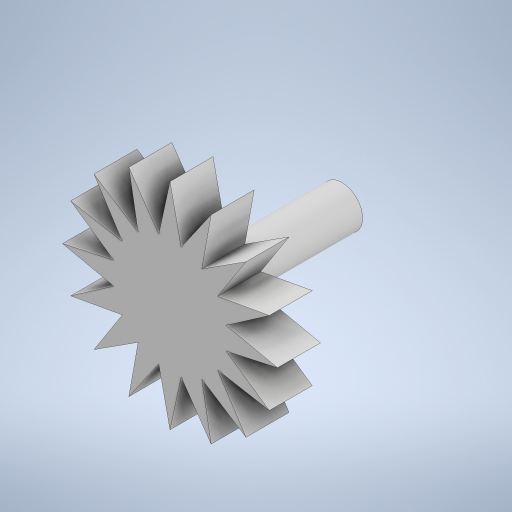
# Autodesk Inventor part: GEAR
Saved by Autodesk Inventor 2024.3 (Build 283343000, 343)
## iProperties
Created: 2024-07-29
Part Number: GEAR
Material: Ogólny
Document SubType Name: Modeling
Designer: User
Density: 1 g/cm^3
Appearance: Domyślna
Author: User
Autodesk Inventor part; units mm, degrees
ref_plane "YZ Plane" through (0, 0, 0) normal (1, 0, 0) x (0, 1, 0)
ref_plane "XZ Plane" through (0, 0, 0) normal (0, 1, 0) x (-1, 0, 0)
ref_plane "XY Plane" through (0, 0, 0) normal (0, 0, 1) x (1, 0, 0)
sketch "Szkic1" plane through (0, 0, 0) normal (0, 0, 1) x (1, 0, 0)
  circle A0 centre (0, 0) radius 3.25
  dimension "d0" = 6.5
  constraints: 1 centre point, 1 coincident
  measures "d0" diameter of A0
extrude "Wyciągnięcie proste1" add sketch "Szkic1" along normal blind 6
sketch "Szkic3" plane through (0, 0, 0) normal (0, 0, -1) x (-1, 0, 0)
  circle A0 centre (0, 0) radius 3.65
  dimension "d11" = 7.3
  constraints: 1 centre point, 1 coincident
  measures "d11" diameter of A0
extrude "Wyciągnięcie proste3" add sketch "Szkic3" against normal blind 6
sketch "Szkic4" plane through (0, 0, 6) normal (0, 0, 1) x (1, 0, 0)
  circle A0 centre (0, 0) radius 3.65 projected
  circle A1 centre (0, 0) radius 3.65
  line L0 (0, 0) -> (0, 9)
  line L1 (0, 9) -> (0, 9.5)
  line L2 (0, 9.5) -> (6.3185, 9.5) construction
  line L3 (0, 9.5) -> (0, 10)
  line L4 (0, 10) -> (1.4493, 3.3499)
  line L5 (0, 10) -> (-1.4493, 3.3499)
  line L6 (-3.8268, 9.2388) -> (0.057, 3.6496)
  line L7 (-3.8268, 9.2388) -> (-2.6209, 2.5403)
  line L8 (-7.0711, 7.0711) -> (-1.344, 3.3936)
  line L9 (-7.0711, 7.0711) -> (-3.3936, 1.344)
  line L10 (-9.2388, 3.8268) -> (-2.5403, 2.6209)
  line L11 (-9.2388, 3.8268) -> (-3.6496, -0.057)
  line L12 (-10, 0) -> (-3.3499, 1.4493)
  line L13 (-10, 0) -> (-3.3499, -1.4493)
  line L14 (-9.2388, -3.8268) -> (-3.6496, 0.057)
  line L15 (-9.2388, -3.8268) -> (-2.5403, -2.6209)
  line L16 (-7.0711, -7.0711) -> (-3.3936, -1.344)
  line L17 (-7.0711, -7.0711) -> (-1.344, -3.3936)
  line L18 (-3.8268, -9.2388) -> (-2.6209, -2.5403)
  line L19 (-3.8268, -9.2388) -> (0.057, -3.6496)
  line L20 (0, -10) -> (-1.4493, -3.3499)
  line L21 (0, -10) -> (1.4493, -3.3499)
  line L22 (3.8268, -9.2388) -> (-0.057, -3.6496)
  line L23 (3.8268, -9.2388) -> (2.6209, -2.5403)
  line L24 (7.0711, -7.0711) -> (1.344, -3.3936)
  line L25 (7.0711, -7.0711) -> (3.3936, -1.344)
  line L26 (9.2388, -3.8268) -> (2.5403, -2.6209)
  line L27 (9.2388, -3.8268) -> (3.6496, 0.057)
  line L28 (10, 0) -> (3.3499, -1.4493)
  line L29 (10, 0) -> (3.3499, 1.4493)
  line L30 (9.2388, 3.8268) -> (3.6496, -0.057)
  line L31 (9.2388, 3.8268) -> (2.5403, 2.6209)
  line L32 (7.0711, 7.0711) -> (3.3936, 1.344)
  line L33 (7.0711, 7.0711) -> (1.344, 3.3936)
  line L34 (3.8268, 9.2388) -> (2.6209, 2.5403)
  line L35 (3.8268, 9.2388) -> (-0.057, 3.6496)
  point P0 (-2.9615, 4.4322)
  point P1 (-4.4322, 2.9615)
  point P2 (-5.2282, 1.0399)
  point P3 (-5.2282, -1.0399)
  point P4 (-4.4322, -2.9615)
  point P5 (-2.9615, -4.4322)
  point P6 (-1.0399, -5.2282)
  point P7 (1.0399, -5.2282)
  point P8 (2.9615, -4.4322)
  point P9 (4.4322, -2.9615)
  point P10 (5.2282, -1.0399)
  point P11 (5.2282, 1.0399)
  point P12 (4.4322, 2.9615)
  point P13 (2.9615, 4.4322)
  point P14 (1.0399, 5.2282)
  point P15 (-1.0399, 5.2282)
  dimension "d34" = 9
  dimension "d39" = 0.5
  dimension "d49" = 0.5
  dimension "d52" = 360
  constraints: 72 end point, 3 vertical, 1 coincident, 1 horizontal, 1 symmetric about line, 85 other
  measures "d34" distance of L0.start L0.end
  measures "d39" distance of L0.end L1.end
  measures "d49" distance of L1.end L3.end
extrude "Wyciągnięcie proste4" add sketch "Szkic4" along normal blind 4
sketch "Szkic5" plane through (0, 0, 0) normal (0, 0, -1) x (-1, 0, 0)
  circle A0 centre (0, 0) radius 3.65
  constraints: 1 centre point, 1 coincident
extrude "Wyciągnięcie proste5" add sketch "Szkic5" along normal blind 6
sketch "Szkic6" plane through (0, 0, -6) normal (0, 0, -1) x (-1, 0, 0)
  circle A0 centre (0, 0) radius 1.425
  circle A1 centre (0, 0) radius 3.65
  dimension "d30" = 2.85
  constraints: 2 centre point, 2 coincident
  measures "d30" diameter of A0
extrude "Wyciągnięcie proste6" cut sketch "Szkic6" against normal blind 12
fillet "Zaokrąglenie1" radius 0.5 1 edges at (1.425, 0, 6)
sketch "Szkic7" plane through (0, 0, -6) normal (0, 0, -1) x (-1, 0, 0)
  circle A0 centre (0, 0) radius 1.925
  dimension "d45" = 3.85
  constraints: 1 centre point, 1 coincident
  measures "d45" diameter of A0
extrude "Wyciągnięcie proste7" add sketch "Szkic7" against normal blind 12.75
fillet "Zaokrąglenie2" radius 0.5 1 edges at (1.925, 0, 6)
